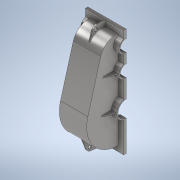
# Autodesk Inventor part: Верх корпуса
Saved by Autodesk Inventor 2022.1 (Build 261234020, 234B)
## iProperties
Created: 2021-12-08
Part Number: Верх корпуса
Material: Сталь, углеродистая
Document SubType Name: Modeling
Designer: GGG
Density: 7.85 g/cm^3
Appearance: С умеренной полировкой
Author: GGG
Autodesk Inventor part; units mm, degrees
ref_plane "YZ Plane" through (0, 0, 0) normal (1, 0, 0) x (0, 1, 0)
ref_plane "XY Plane" through (0, 0, 0) normal (0, 0, 1) x (1, 0, 0)
sketch "Эскиз1" plane through (0, 0, 0) normal (0, 0, 1) x (1, 0, 0)
  line L0 (-175, -493) -> (175, -493)
  line L1 (175, -493) -> (175, 493)
  line L2 (175, 493) -> (-175, 493)
  line L3 (-175, 493) -> (-175, -493)
  line L4 (-175, -493) -> (175, 493) construction
  line L5 (175, -493) -> (-175, 493) construction
  point P0 (0, 0)
  dimension "d0" = 350
  dimension "d1" = 986
  constraints: 12 end point, 2 midpoint, 2 parallel, 1 horizontal, 1 perpendicular
  measures "d0" distance of L1.end L2.end
  measures "d1" distance of L0.end L1.end
extrude "Выдавливание1" add sketch "Эскиз1" along normal blind 22.5
sketch "Эскиз2" plane through (0, 0, 0) normal (1, 0, 0) x (0, 1, 0)
  line L0 (493, 22.5) -> (-493, 22.5) projected
  point P0 (0, 0)
sketch "Эскиз3" plane through (0, 0, 0) normal (1, 0, 0) x (0, 1, 0)
  line L0 (493, 22.5) -> (-493, 22.5) construction
  line L1 (-154.4, 22.5) -> (-154.4, 0) construction
  line L2 (493, 0) -> (-493, 0) construction
  line L3 (-493, 0) -> (-493, 22.5) construction
  arc A0 (-76.2115, 300.5144) -> (-443.2, 22.5) centre (-154.4, 22.5) ccw
  line L4 (443.2, 0) -> (443.2, 22.5) construction
  line L5 (493, 0) -> (493, 22.5) construction
  arc A1 (443.2, 22.5) -> (342.1044, 182.8676) centre (300.1045, 44.3418) ccw
  line L6 (-443.2, 22.5) -> (443.2, 22.5)
  line L7 (-76.2115, 300.5144) -> (342.1044, 182.8676)
  point P0 (0, 0)
  point P1 (342.1044, 182.8676)
  dimension "d4" = 338.6
  dimension "d6" = 288.8
  dimension "d7" = 49.8
  constraints: 8 end point, 5 point on line, 4 point on circle, 3 coincident, 2 centre point, 1 collinear, 1 perpendicular, 1 tangent, 1 vertical
  measures "d4" distance between parallel lines of L3 L1
  measures "d6" radius of A0
  measures "d7" distance between parallel lines of L5 L4
extrude "Выдавливание2" add sketch "Эскиз3" along normal mid plane 250.2
shell "Оболочка1" thickness 6 removed faces 1 at (58.3333, -164.3333, 0)
sketch "Эскиз6" plane through (0, 0, 0) normal (1, 0, 0) x (0, 1, 0)
  line L0 (493, 0) -> (493, 22.5) projected
  line L1 (493, 22.5) -> (493, 90.7866)
  line L2 (338.5372, 177.6836) -> (458.5875, 138.2948)
  arc A0 (493, 90.7866) -> (458.5875, 138.2948) centre (443, 90.7866) ccw
  circle A1 centre (458.5875, 107.6076) radius 15
  point P0 (0, 0)
  point P1 (443.2, 22.5)
  dimension "d14" = 50
  dimension "d28" = 30
  constraints: 4 end point, 2 centre point, 2 point on circle, 2 tangent, 1 vertical
  measures "d14" radius of A0
  measures "d28" diameter of A1
extrude "Ребро жесткости1" add sketch "Эскиз6" along normal mid plane 10 rib yes fills toward (492.95, 11.25) open curves L0 L1 A0 L2
sketch "Эскиз7" plane through (0, 0, 0) normal (1, 0, 0) x (0, 1, 0)
  line L0 (-493, 0) -> (-493, 22.5) projected
  line L1 (-493, 22.5) -> (-479.9014, 152.7174)
  line L2 (-448.1609, 194.3574) -> (-354.8911, 230.3672)
  arc A0 (-76.2115, 300.5144) -> (-443.2, 22.5) centre (-154.4, 22.5) ccw projected
  arc A1 (-448.1609, 194.3574) -> (-479.9014, 152.7174) centre (-430.1524, 147.7131) ccw
  circle A2 centre (-448.1609, 160.2174) radius 15
  point P0 (0, 0)
  dimension "d21" = 50
  dimension "d31" = 30
  constraints: 4 end point, 3 point on circle, 2 centre point, 2 tangent
  measures "d21" radius of A1
  measures "d31" diameter of A2
extrude "Ребро жесткости2" add sketch "Эскиз7" along normal mid plane 10 rib yes fills toward (-492.95, 11.25) open curves L0 L1 A1 L2
extrude "Выдавливание3" cut sketch "Эскиз6" along normal mid plane 55.25
extrude "Выдавливание4" cut sketch "Эскиз7" along normal mid plane 32.75
sketch "Эскиз8" plane through (125.1, 0, 0) normal (1, 0, 0) x (0, 0, -1)
  line L0 (0, 487) -> (0, -487) projected
  line L1 (0, 493) -> (-22.5, 493) projected
  circle A0 centre (0, 363) radius 55
  circle A1 centre (0, 163) radius 55
  circle A2 centre (0, -137) radius 75
  circle A3 centre (0, -137) radius 86.25
  circle A4 centre (0, 163) radius 66.25
  circle A5 centre (0, 363) radius 66.25
  point P0 (0, 0)
  point P1 (0, 429.25)
  point P2 (0, 296.75)
  point P3 (0, 308)
  point P4 (0, 418)
  point P5 (0, 229.25)
  point P6 (0, 96.75)
  point P7 (0, 108)
  point P8 (0, 218)
  point P9 (0, -50.75)
  point P10 (0, -223.25)
  point P11 (0, -212)
  point P12 (0, -62)
  dimension "d34" = 130
  dimension "d35" = 200
  dimension "d36" = 300
  dimension "d53" = 110
  dimension "d54" = 132.5
  dimension "d55" = 110
  dimension "d56" = 132.5
  dimension "d57" = 150
  dimension "d58" = 172.5
  constraints: 6 centre point, 6 coincident, 3 point on line
  measures "d34" distance from line of L1 point (0, 363)
  measures "d35" distance of point (0, 363) point (0, 163)
  measures "d36" distance of point (0, 163) point (0, -137)
  measures "d53" diameter of A0
  measures "d54" diameter of A5
  measures "d55" diameter of A1
  measures "d56" diameter of A4
  measures "d57" diameter of A2
  measures "d58" diameter of A3
sketch "Эскиз14" plane through (0, 0, 0) normal (0, 0, -1) x (-1, 0, 0)
  line L0 (-119.1, -437.1363) -> (119.1, -437.1363) projected
  line L1 (-119.1, 436.0353) -> (-119.1, -437.1363) projected
  line L2 (119.1, 436.0353) -> (-119.1, 436.0353) projected
  line L3 (119.1, -437.1363) -> (119.1, 436.0353) projected
  line L4 (-169, -487) -> (-169, 487) projected
  line L5 (169, -487) -> (-169, -487) projected
  line L6 (169, 487) -> (169, -487) projected
  line L7 (-169, 487) -> (169, 487) projected
  point P0 (0, 0)
extrude "Выдавливание18" add sketch "Эскиз14" against normal blind 20
extrude "Выдавливание19" add sketch "Эскиз8" along normal up to surface (49.9 mm away) contours L0 A0 A5 | L0 A1 A4 | L0 A2 A3 picked at (-62.2709, 364.6916) picked at (-62.2709, 164.6916) picked at (-4.285, -54.8211)
extrude "Выдавливание20" cut sketch "Эскиз8" along normal mid plane 1012.75 contours A0 L0 | L0 A0 | A1 L0 | L0 A1 | A2 L0 | L0 A2
sketch "Эскиз15" plane through (-125.1, 0, 0) normal (-1, 0, 0) x (0, 0, 1)
  arc A0 (22.5, 300.6878) -> (22.5, 425.3122) centre (0, 363) ccw projected
  arc A1 (22.5, 312.8129) -> (22.5, 413.1871) centre (0, 363) ccw projected
  arc A2 (22.5, 112.8129) -> (22.5, 213.1871) centre (0, 163) ccw projected
  arc A3 (22.5, 100.6878) -> (22.5, 225.3122) centre (0, 163) ccw projected
  arc A4 (22.5, -208.5454) -> (22.5, -65.4546) centre (0, -137) ccw projected
  arc A5 (22.5, -220.2635) -> (22.5, -53.7365) centre (0, -137) ccw projected
  line L0 (22.5, 112.8129) -> (22.5, -65.4546) projected
  line L1 (22.5, 493) -> (22.5, 443.2) projected
  line L2 (22.5, 443.2) -> (22.5, 413.1871) projected
  arc A6 (22.5, 413.1871) -> (0, 418) centre (0, 363) ccw projected
  line L3 (0, 418) -> (0, 493) projected
  line L4 (0, 493) -> (22.5, 493) projected
  arc A7 (182.8676, 342.1044) -> (22.5, 443.2) centre (44.3418, 300.1045) ccw projected
  line L5 (182.8676, 342.1044) -> (300.5144, -76.2115) projected
  arc A8 (22.5, -443.2) -> (300.5144, -76.2115) centre (22.5, -154.4) ccw projected
  line L6 (22.5, -443.2) -> (22.5, -493) projected
  line L7 (22.5, -493) -> (0, -493) projected
  line L8 (0, -493) -> (0, -212) projected
  arc A9 (0, -212) -> (22.5, -208.5454) centre (0, -137) ccw projected
  line L9 (22.5, -208.5454) -> (22.5, -443.2) projected
  arc A10 (22.5, 312.8129) -> (22.5, 413.1871) centre (0, 363) ccw projected
  arc A11 (0, 308) -> (22.5, 312.8129) centre (0, 363) ccw projected
  line L10 (0, 218) -> (0, 308) projected
  arc A12 (22.5, 213.1871) -> (0, 218) centre (0, 163) ccw projected
  arc A13 (22.5, 112.8129) -> (22.5, 213.1871) centre (0, 163) ccw projected
  arc A14 (0, 108) -> (22.5, 112.8129) centre (0, 163) ccw projected
  line L11 (0, -62) -> (0, 108) projected
  arc A15 (22.5, -65.4546) -> (0, -62) centre (0, -137) ccw projected
  line L12 (22.5, 112.8129) -> (22.5, -65.4546) projected
  arc A16 (22.5, -208.5454) -> (22.5, -65.4546) centre (0, -137) ccw projected
  line L13 (22.5, 312.8129) -> (22.5, 213.1871) projected
  arc A17 (0, 308) -> (22.5, 312.8129) centre (0, 363) ccw projected
  arc A18 (22.5, 413.1871) -> (0, 418) centre (0, 363) ccw projected
  circle A19 centre (0, 363) radius 66.25 projected
  arc A20 (22.5, 213.1871) -> (0, 218) centre (0, 163) ccw projected
  arc A21 (0, 108) -> (22.5, 112.8129) centre (0, 163) ccw projected
  arc A22 (0, -212) -> (22.5, -208.5454) centre (0, -137) ccw projected
  arc A23 (22.5, -65.4546) -> (0, -62) centre (0, -137) ccw projected
  line L14 (22.5, -208.5454) -> (22.5, -493) projected
  line L15 (22.5, 312.8129) -> (22.5, 213.1871) projected
  line L16 (22.5, 493) -> (22.5, 413.1871) projected
  point P0 (0, 0)
extrude "Выдавливание21" add sketch "Эскиз15" along normal up to surface (49.9 mm away) contours L13 A1 L2 A0 | A3 L0 A2 L13 | A5 L9 A4 L0
ref_plane "РабПлоскость1" through (0, -136.5, 0) normal (0, 1, 0) x (-1, 0, 0)
ref_plane "РабПлоскость2" through (0, 164, 0) normal (0, 1, 0) x (-1, 0, 0)
sketch "Эскиз16" plane through (0, -136.5, 0) normal (0, 1, 0) x (-1, 0, 0)
  line L0 (-123.7926, 179.6448) -> (-167.2431, 86.25)
  line L1 (-125.1, 86.25) -> (-175, 86.25) projected
  point P0 (0, 0)
  constraints: 2 end point, 1 point on line
extrude "Ребро жесткости3" add sketch "Эскиз16" along normal mid plane 10 rib yes fills toward (-145.4725, 132.9263) open curves L0
sketch "Эскиз17" plane through (0, 164, 0) normal (0, 1, 0) x (-1, 0, 0)
  line L0 (-166.5576, 67.2346) -> (-119.1, 178.8052)
  line L1 (-119.1, 177.1083) -> (-119.1, 294.7385) projected
  point P0 (0, 0)
  constraints: 2 end point, 1 point on line
extrude "Ребро жесткости4" add sketch "Эскиз17" along normal mid plane 10 rib yes fills toward (-142.7828, 123.0003) open curves L0
mirror "Зеркальное отражение1" about plane through (0, 0, 0) normal (1, 0, 0) of "Ребро жесткости4", "Ребро жесткости3"
